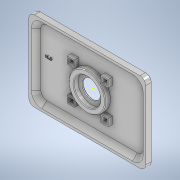
# Autodesk Inventor part: StageInsert_Inserts_v1.2
Saved by Autodesk Inventor 2026 (Build 300175050, 175E)
## iProperties
Created: 2024-02-02
Part Number: StageInsert_Inserts_v1.2
Material: PC/ABS-Kunststoff
Document SubType Name: Modeling
Designer: neuhau0004
Density: 0.357273 g/cm^3
Appearance: Aluminium - poliert
Author: neuhau0004
Autodesk Inventor part; units mm, degrees
ref_plane "YZ Plane" through (0, 0, 0) normal (1, 0, 0) x (0, 1, 0)
ref_plane "XZ Plane" through (0, 0, 0) normal (0, 1, 0) x (-1, 0, 0)
ref_plane "XY Plane" through (0, 0, 0) normal (0, 0, 1) x (1, 0, 0)
sketch "Skizze2" plane through (0, 0, 0) normal (0, 0, 1) x (1, 0, 0)
  line L0 (-71.875, 54.85) -> (71.875, 54.85)
  line L1 (79.875, 46.85) -> (79.875, -46.85)
  line L2 (71.875, -54.85) -> (-71.875, -54.85)
  line L3 (-79.875, -46.85) -> (-79.875, 46.85)
  line L4 (-79.875, 54.85) -> (79.875, -54.85) construction
  line L5 (79.875, 54.85) -> (-79.875, -54.85) construction
  arc A0 (-71.875, 54.85) -> (-79.875, 46.85) centre (-71.875, 46.85) ccw
  arc A1 (-79.875, -46.85) -> (-71.875, -54.85) centre (-71.875, -46.85) ccw
  arc A2 (79.875, 46.85) -> (71.875, 54.85) centre (71.875, 46.85) ccw
  arc A3 (71.875, -54.85) -> (79.875, -46.85) centre (71.875, -46.85) ccw
  line L6 (-61.75, 44.75) -> (61.75, 44.75)
  line L7 (69.75, 36.75) -> (69.75, -36.75)
  line L8 (61.75, -44.75) -> (-61.75, -44.75)
  line L9 (-69.75, -36.75) -> (-69.75, 36.75)
  line L10 (-69.75, 44.75) -> (69.75, -44.75) construction
  line L11 (69.75, 44.75) -> (-69.75, -44.75) construction
  arc A4 (-61.75, 44.75) -> (-69.75, 36.75) centre (-61.75, 36.75) ccw
  arc A5 (-69.75, -36.75) -> (-61.75, -44.75) centre (-61.75, -36.75) ccw
  arc A6 (61.75, -44.75) -> (69.75, -36.75) centre (61.75, -36.75) ccw
  arc A7 (69.75, 36.75) -> (61.75, 44.75) centre (61.75, 36.75) ccw
  point P0 (0, 0)
  point P1 (0, 0)
  point P2 (-77.5, -10)
  point P3 (77.5, 10)
  point P4 (0, 52.5)
  point P5 (0, -52.5)
  dimension "d0" = 159.75
  dimension "d1" = 109.7
  dimension "d2" = 8
  dimension "d3" = 139.5
  dimension "d4" = 89.5
  dimension "d5" = 8
  dimension "d24" = 105
  dimension "d25" = 10
  dimension "d26" = 10
  constraints: 24 end point, 16 point on circle, 16 point on line, 16 tangent, 8 centre point, 6 equal radius, 4 midpoint, 4 parallel, 2 horizontal, 2 perpendicular, 1 coincident
  measures "d0" distance of L4.end L5.end
  measures "d1" distance of L5.start L4.end
  measures "d2" radius of A0
  measures "d3" distance of L10.end L11.end
  measures "d4" distance of L11.start L10.end
  measures "d5" radius of A4
  measures "d24" distance of point (0, -52.5) point (0, 52.5)
  measures "d25" vertical distance of point (0, 0) point (77.5, 10)
  measures "d26" vertical distance of point (-77.5, -10) point (0, 0)
extrude "Extrusion1" add sketch "Skizze2" along normal blind 8
hole "Bohrung1" [suppressed]
sketch "Skizze3" plane through (0, 0, 0) normal (0, 0, -1) x (-1, 0, 0)
  line L0 (69.8, -50.8) -> (-69.8, -50.8)
  line L1 (-75.8, -44.8) -> (-75.8, 44.8)
  line L2 (-69.8, 50.8) -> (69.8, 50.8)
  line L3 (75.8, 44.8) -> (75.8, -44.8)
  line L4 (75.8, -50.8) -> (-75.8, 50.8) construction
  line L5 (-75.8, -50.8) -> (75.8, 50.8) construction
  arc A0 (69.8, -50.8) -> (75.8, -44.8) centre (69.8, -44.8) ccw
  arc A1 (75.8, 44.8) -> (69.8, 50.8) centre (69.8, 44.8) ccw
  arc A2 (-69.8, 50.8) -> (-75.8, 44.8) centre (-69.8, 44.8) ccw
  arc A3 (-75.8, -44.8) -> (-69.8, -50.8) centre (-69.8, -44.8) ccw
  line L6 (89.8749, -63.3086) -> (-89.8749, -63.3086)
  line L7 (-89.8749, -63.3086) -> (-89.8749, 63.3086)
  line L8 (-89.8749, 63.3086) -> (89.8749, 63.3086)
  line L9 (89.8749, 63.3086) -> (89.8749, -63.3086)
  line L10 (89.8749, -63.3086) -> (-89.8749, 63.3086) construction
  line L11 (-89.8749, -63.3086) -> (89.8749, 63.3086) construction
  line L12 (39.5, -33) -> (-39.5, -33)
  line L13 (-42.5, -30) -> (-42.5, 30)
  line L14 (-39.5, 33) -> (39.5, 33)
  line L15 (42.5, 30) -> (42.5, -30)
  line L16 (42.5, -33) -> (-42.5, 33) construction
  line L17 (-42.5, -33) -> (42.5, 33) construction
  arc A4 (39.5, -33) -> (42.5, -30) centre (39.5, -30) ccw
  arc A5 (42.5, 30) -> (39.5, 33) centre (39.5, 30) ccw
  arc A6 (-42.5, -30) -> (-39.5, -33) centre (-39.5, -30) ccw
  arc A7 (-39.5, 33) -> (-42.5, 30) centre (-39.5, 30) ccw
  circle A8 centre (0, 0) radius 12.5
  circle A9 centre (0, 0) radius 18.5
  dimension "d18" = 151.6
  dimension "d19" = 101.6
  dimension "d20" = 6
  dimension "d30" = 85
  dimension "d31" = 66
  dimension "d32" = 3
  dimension "d39" = 3
  dimension "d40" = 25
  dimension "d41" = 37
  constraints: 36 end point, 16 point on circle, 16 point on line, 16 tangent, 10 centre point, 7 midpoint, 6 equal radius, 6 parallel, 3 horizontal, 3 perpendicular, 2 coincident
  measures "d18" distance of L4.end L5.end
  measures "d19" distance of L5.start L4.end
  measures "d20" radius of A0
  measures "d30" distance of L16.end L17.end
  measures "d31" distance of L17.start L16.end
  measures "d32" radius of A4
  measures "d39" radius of A7
  measures "d40" diameter of A8
  measures "d41" diameter of A9
extrude "Extrusion2" [suppressed]
extrude "Extrusion4" add sketch "Skizze3" against normal blind 1.5 contours L0 A3 L1 A2 L2 A1 L3 A0 | L12 A6 L13 A7 L14 A5 L15 A4 | A9
draft "Flächenverjüngung3" angle 45 pull direction (0, 0, 1) fixed plane through (50.6667, 0, 1.5) normal (0, 0, 1) faces at (-20.5833, 44.75, 3.6667) (67.1914, 42.6144, 5.8333) (-67.1914, 42.6144, 5.8333) (69.75, 12.25, 5.8333) (-69.75, -12.25, 5.8333) (67.6144, -42.1914, 5.8333) (-69.197, -39.6727, 5.8333) (20.5833, -44.75, 5.8333)
sketch "Skizze5" plane through (0, 0, 1.5) normal (0, 0, 1) x (1, 0, 0)
  circle A0 centre (0, 0) radius 18
  circle A1 centre (0, 0) radius 25
  dimension "d42" = 36
  dimension "d43" = 50
  constraints: 2 centre point, 2 coincident
  measures "d42" diameter of A0
  measures "d43" diameter of A1
extrude "Extrusion5" add sketch "Skizze5" along normal blind 7
sketch "Skizze6" plane through (0, 0, 1.5) normal (0, 0, 1) x (1, 0, 0)
  circle A0 centre (0, 0) radius 12.5
  circle A1 centre (0, 0) radius 18.5
  constraints: 2 centre point, 2 coincident
extrude "Extrusion6" add sketch "Skizze6" along normal blind 1
chamfer "Fase2" distance 1 angle 45 3 edges at (-18, 0, 8.5) (-25, 0, 8.5) (12.5, 0, 0)
feature "Verdickung1" [suppressed]
sketch "Skizze7" plane through (0, 0, 1.5) normal (0, 0, 1) x (1, 0, 0)
  line L0 (-26.525, 26.525) -> (-19.475, 26.525)
  line L1 (-19.475, 26.525) -> (-19.475, 19.475)
  line L2 (-19.475, 19.475) -> (-26.525, 19.475)
  line L3 (-26.525, 19.475) -> (-26.525, 26.525)
  line L4 (-26.525, 26.525) -> (-19.475, 19.475) construction
  line L5 (-19.475, 26.525) -> (-26.525, 19.475) construction
  line L6 (-28, 28) -> (-18, 28)
  line L7 (-18, 28) -> (-18, 18)
  line L8 (-18, 18) -> (-28, 18)
  line L9 (-28, 18) -> (-28, 28)
  line L10 (-28, 28) -> (-18, 18) construction
  line L11 (-18, 28) -> (-28, 18) construction
  line L12 (19.475, 26.525) -> (26.525, 26.525)
  line L13 (26.525, 26.525) -> (26.525, 19.475)
  line L14 (26.525, 19.475) -> (19.475, 19.475)
  line L15 (19.475, 19.475) -> (19.475, 26.525)
  line L16 (19.475, 26.525) -> (26.525, 19.475) construction
  line L17 (26.525, 26.525) -> (19.475, 19.475) construction
  line L18 (18, 28) -> (28, 28)
  line L19 (28, 28) -> (28, 18)
  line L20 (28, 18) -> (18, 18)
  line L21 (18, 18) -> (18, 28)
  line L22 (18, 28) -> (28, 18) construction
  line L23 (28, 28) -> (18, 18) construction
  line L24 (-26.525, -19.475) -> (-19.475, -19.475)
  line L25 (-19.475, -19.475) -> (-19.475, -26.525)
  line L26 (-19.475, -26.525) -> (-26.525, -26.525)
  line L27 (-26.525, -26.525) -> (-26.525, -19.475)
  line L28 (-26.525, -19.475) -> (-19.475, -26.525) construction
  line L29 (-19.475, -19.475) -> (-26.525, -26.525) construction
  line L30 (-28, -18) -> (-18, -18)
  line L31 (-18, -18) -> (-18, -28)
  line L32 (-18, -28) -> (-28, -28)
  line L33 (-28, -28) -> (-28, -18)
  line L34 (-28, -18) -> (-18, -28) construction
  line L35 (-18, -18) -> (-28, -28) construction
  line L36 (19.475, -19.475) -> (26.525, -19.475)
  line L37 (26.525, -19.475) -> (26.525, -26.525)
  line L38 (26.525, -26.525) -> (19.475, -26.525)
  line L39 (19.475, -26.525) -> (19.475, -19.475)
  line L40 (19.475, -19.475) -> (26.525, -26.525) construction
  line L41 (26.525, -19.475) -> (19.475, -26.525) construction
  line L42 (18, -18) -> (28, -18)
  line L43 (28, -18) -> (28, -28)
  line L44 (28, -28) -> (18, -28)
  line L45 (18, -28) -> (18, -18)
  line L46 (18, -18) -> (28, -28) construction
  line L47 (28, -18) -> (18, -28) construction
  point P0 (0, 0)
  point P1 (-23, 23)
  point P2 (25, -25)
  point P3 (-25, -25)
  point P4 (23, 23)
  point P5 (-23, -23)
  point P6 (23, -23)
  dimension "d53" = 7.05
  dimension "d54" = 7.05
  dimension "d55" = 10
  dimension "d56" = 10
  dimension "d72" = 23
  dimension "d75" = 46
  dimension "d78" = 46
  dimension "d81" = 23
  constraints: 96 end point, 16 midpoint, 4 parallel, 3 horizontal, 2 collinear, 2 perpendicular, 1 vertical, 61 other
  measures "d53" distance of L1.end L2.end
  measures "d54" distance of L0.end L1.end
  measures "d55" distance of L7.end L8.end
  measures "d56" distance of L6.end L7.end
  measures "d72" horizontal distance of point (0, 0) point (-23, 23)
  measures "d75" distance of L0.start L12.start
  measures "d78" distance of L0.start L24.start
  measures "d81" horizontal distance of point (0, 0) point (-23, 23)
extrude "Extrusion7" add sketch "Skizze7" along normal blind 6
thicken "Verdickung2" operation add thickness 0.2 both sides no extend neighbours yes toward (-1, 0, 0) faces at (79.875, -15.6167, 2.6667) (77.3164, -52.7144, 5.3333) (-23.9583, -54.85, 2.6667) (-77.7394, -52.2914, 5.3333) (77.3164, 52.7144, 5.3333) (23.9583, 54.85, 2.6667) (-79.8526, 47.4478, 5.3333) (-79.875, 15.6167, 2.6667)
sketch "Skizze8" plane through (0, 0, 1.5) normal (0, 0, 1) x (1, 0, 0)
  line L0 (-63.1236, 9.75) -> (-54.0162, 9.75) construction
  line L1 (-54.0162, 9.75) -> (-54.0162, 6.1053) construction
  line L2 (-54.0162, 6.1053) -> (-63.1236, 6.1053) construction
  line L3 (-63.1236, 6.1053) -> (-63.1236, 9.75) construction
  line L4 (-61.75, 44.75) -> (61.75, 44.75) projected
  line L5 (-60.7411, 8.8027) -> (-61.731, 6.1763)
  line L6 (-61.731, 6.1763) -> (-62.1281, 6.1763)
  line L7 (-62.1281, 6.1763) -> (-63.1094, 8.8027)
  line L8 (-63.1094, 8.8027) -> (-62.6301, 8.8027)
  line L9 (-62.6301, 8.8027) -> (-61.9125, 6.7804)
  line L10 (-61.9125, 6.7804) -> (-61.2006, 8.8027)
  line L11 (-61.2006, 8.8027) -> (-60.7411, 8.8027)
  line L12 (-58.4891, 6.1763) -> (-60.1966, 6.1763)
  line L13 (-60.1966, 6.1763) -> (-60.1966, 6.5336)
  line L14 (-60.1966, 6.5336) -> (-59.5612, 6.5336)
  line L15 (-59.5612, 6.5336) -> (-59.5612, 8.8793)
  line L16 (-59.5612, 8.8793) -> (-60.1966, 8.8793)
  line L17 (-60.1966, 8.8793) -> (-60.1966, 9.1998)
  spline S0 degree 2 poles (-60.1966, 9.1998) (-59.8363, 9.1998) (-59.496, 9.404) (-59.4733, 9.6876) knots 0 0 0 1 2 2 2
  line L18 (-59.4733, 9.6876) -> (-59.1103, 9.6876)
  line L19 (-59.1103, 9.6876) -> (-59.1103, 6.5336)
  line L20 (-59.1103, 6.5336) -> (-58.4891, 6.5336)
  line L21 (-58.4891, 6.5336) -> (-58.4891, 6.1763)
  line L22 (-57.0936, 6.1763) -> (-57.6552, 6.1763)
  line L23 (-57.6552, 6.1763) -> (-57.6552, 6.8456)
  line L24 (-57.6552, 6.8456) -> (-57.0936, 6.8456)
  line L25 (-57.0936, 6.8456) -> (-57.0936, 6.1763)
  spline S1 degree 2 poles (-55.4429, 9.3444) (-55.5705, 9.3444) (-55.823, 9.282) (-55.9449, 9.2338) knots 0 0 0 1 2 2 2
  spline S2 degree 2 poles (-55.9449, 9.2338) (-56.0584, 9.1856) (-56.2257, 9.0835) (-56.291, 9.0381) knots 0 0 0 1 2 2 2
  line L26 (-56.291, 9.0381) -> (-56.3193, 9.0381)
  line L27 (-56.3193, 9.0381) -> (-56.3193, 9.5344)
  spline S3 degree 2 poles (-56.3193, 9.5344) (-56.1662, 9.6167) (-55.6415, 9.75) (-55.406, 9.75) knots 0 0 0 1 2 2 2
  spline S4 degree 2 poles (-55.406, 9.75) (-55.1678, 9.75) (-54.8133, 9.6536) (-54.6686, 9.5515) knots 0 0 0 1 2 2 2
  spline S5 degree 2 poles (-54.6686, 9.5515) (-54.5154, 9.4408) (-54.3566, 9.1203) (-54.3566, 8.9048) knots 0 0 0 1 2 2 2
  spline S6 degree 2 poles (-54.3566, 8.9048) (-54.3566, 8.6155) (-54.7367, 8.1787) (-55.0033, 8.122) knots 0 0 0 1 2 2 2
  line L28 (-55.0033, 8.122) -> (-55.0033, 8.0879)
  spline S7 degree 2 poles (-55.0033, 8.0879) (-54.8927, 8.0652) (-54.6402, 7.9631) (-54.5325, 7.861) knots 0 0 0 1 2 2 2
  spline S8 degree 2 poles (-54.5325, 7.861) (-54.4247, 7.7618) (-54.2885, 7.4441) (-54.2885, 7.2143) knots 0 0 0 1 2 2 2
  spline S9 degree 2 poles (-54.2885, 7.2143) (-54.2885, 6.9789) (-54.4502, 6.579) (-54.5977, 6.4259) knots 0 0 0 1 2 2 2
  spline S10 degree 2 poles (-54.5977, 6.4259) (-54.7509, 6.267) (-55.1848, 6.1025) (-55.4599, 6.1025) knots 0 0 0 1 2 2 2
  spline S11 degree 2 poles (-55.4599, 6.1025) (-55.7237, 6.1025) (-56.2399, 6.2301) (-56.4158, 6.3181) knots 0 0 0 1 2 2 2
  line L29 (-56.4158, 6.3181) -> (-56.4158, 6.8144)
  line L30 (-56.4158, 6.8144) -> (-56.3817, 6.8144)
  spline S12 degree 2 poles (-56.3817, 6.8144) (-56.2342, 6.7066) (-55.735, 6.5081) (-55.4883, 6.5081) knots 0 0 0 1 2 2 2
  spline S13 degree 2 poles (-55.4883, 6.5081) (-55.3436, 6.5081) (-55.0543, 6.5989) (-54.9579, 6.7038) knots 0 0 0 1 2 2 2
  spline S14 degree 2 poles (-54.9579, 6.7038) (-54.8643, 6.8088) (-54.765, 7.0583) (-54.765, 7.2484) knots 0 0 0 1 2 2 2
  spline S15 degree 2 poles (-54.765, 7.2484) (-54.765, 7.4384) (-54.8756, 7.6852) (-54.9749, 7.7561) knots 0 0 0 1 2 2 2
  spline S16 degree 2 poles (-54.9749, 7.7561) (-55.0742, 7.827) (-55.3436, 7.8809) (-55.5025, 7.8809) knots 0 0 0 1 2 2 2
  line L31 (-55.5025, 7.8809) -> (-55.701, 7.8809)
  line L32 (-55.701, 7.8809) -> (-55.701, 8.2694)
  line L33 (-55.701, 8.2694) -> (-55.545, 8.2694)
  spline S17 degree 2 poles (-55.545, 8.2694) (-55.2302, 8.2694) (-54.8331, 8.5701) (-54.8331, 8.8566) knots 0 0 0 1 2 2 2
  spline S18 degree 2 poles (-54.8331, 8.8566) (-54.8331, 8.9899) (-54.9352, 9.1799) (-55.0175, 9.2366) knots 0 0 0 1 2 2 2
  spline S19 degree 2 poles (-55.0175, 9.2366) (-55.1054, 9.2962) (-55.3209, 9.3444) (-55.4429, 9.3444) knots 0 0 0 1 2 2 2
  point P0 (0, 0)
  dimension "d84" = 35
  constraints: 2 other
  measures "d84" distance between parallel lines of L4 L0
emboss "Prägen1" sketch "Skizze8" operation add depth 1 direction (0, 0, -1)
sketch "Skizze10" plane through (0, 0, 1.5) normal (0, 0, 1) x (1, 0, 0)
  point P0 (0, 0)
extrude "Extrusion8" cut sketch "Skizze7" against normal blind 0.5 contours L0 L1 L2 L3 | L12 L13 L14 L15 | L24 L25 L26 L27 | L36 L37 L38 L39
chamfer "Fase3" distance 0.5 angle 45 8 edges at (0, -54.65, 0) (77.3904, -52.3654, 0) (79.675, 0, 0) (77.3904, 52.3654, 0) (0, 54.65, 0) (-77.3904, 52.3654, 0) (-79.675, 0, 0) (-77.3904, -52.3654, 0)
